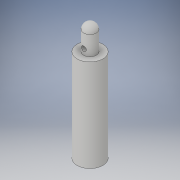
# Autodesk Inventor part: whiteNip
Saved by Autodesk Inventor 2017 (Build 210142000, 142)
## iProperties
Created: 2017-02-17
Part Number: whiteNip
Material: Generic
Document SubType Name: Modeling
Designer: kingb
Density: 1 g/cm^3
Appearance: Default
Author: kingb
Autodesk Inventor part; units mm, degrees
ref_plane "YZ Plane" through (0, 0, 0) normal (1, 0, 0) x (0, 1, 0)
ref_plane "XZ Plane" through (0, 0, 0) normal (0, 1, 0) x (-1, 0, 0)
sketch "Sketch1" plane through (0, 0, 0) normal (0, 1, 0) x (-1, 0, 0)
  circle A0 centre (0, 0) radius 6.35
  dimension "d0" = 12.7
  constraints: 1 centre point, 1 coincident
  measures "d0" diameter of A0
extrude "Extrusion1" add sketch "Sketch1" along normal blind 45.72
sketch "Sketch2" plane through (0, 45.72, 0) normal (0, 1, 0) x (1, 0, 0)
  circle A0 centre (0, 0) radius 3.175
  dimension "d3" = 6.35
  constraints: 1 centre point, 1 coincident
  measures "d3" diameter of A0
extrude "Extrusion2" add sketch "Sketch2" along normal blind 12.7
ref_plane "Work Plane1" through (0, 45.72, 3.175) normal (0, 0, 1) x (1, 0, 0)
sketch "Sketch3" plane through (0, 45.72, 3.175) normal (0, 0, 1) x (1, 0, 0)
  circle A0 centre (0, 2.7781) radius 1.1906
  line L0 (-3.175, 0) -> (-3.175, 12.7) projected
  line L1 (-3.175, 1.5875) -> (3.175, 1.5875)
  line L2 (3.175, 0) -> (3.175, 12.7) projected
  line L3 (6.35, 0) -> (-6.35, 0) projected
  point P0 (0, -45.72)
  dimension "d6" = 2.3813
  dimension "d7" = 1.5875
  constraints: 2 end point, 2 point on line, 1 centre point, 1 horizontal, 1 tangent
  measures "d6" diameter of A0
  measures "d7" distance between parallel lines of L3 L1
extrude "Extrusion3" cut sketch "Sketch3" against normal up to next contours A0
sketch "Sketch4" plane through (0, 0, 0) normal (0, -1, 0) x (1, 0, 0)
  point P0 (0, 0)
  point P1 (0, 0)
  constraints: 1 coincident
hole "Hole1" at (0, 0, 0) at (0, 0, 0) direction (0, 1, 0) diameter 2.54 depth 28.321
fillet "Fillet1" radius 3.175 1 edges at (-3.175, 58.42, 0)
body "Solid1"
